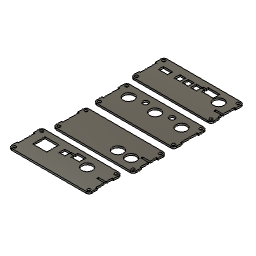
BlinkBoxEndV2v5 (Autodesk Fusion 360 design; units mm, degrees)
Autodesk Fusion 360 part; units mm, degrees
sketch "FrontSketch" plane through (0, 0, 0) normal (0, 1, 0) x (1, 0, 0)
  line L0 (0, 0) -> (92, 0) construction
  line L1 (0, 0) -> (-2.45, 0) construction
  line L2 (94.45, 0) -> (92, 0) construction
  line L3 (-2.45, 8) -> (94.45, 8) construction
  line L4 (94.45, 8) -> (94.45, -31.9) construction
  line L5 (94.45, -31.9) -> (-2.45, -31.9) construction
  line L6 (-2.45, -31.9) -> (-2.45, 8) construction
  line L7 (-2.45, -28.4) -> (1.05, -28.4) construction
  line L8 (1.05, -28.4) -> (1.05, -31.9) construction
  circle A0 centre (1.05, -28.4) radius 1.825
  arc A1 (-2.45, -28.4) -> (1.05, -31.9) centre (1.05, -28.4) ccw
  line L9 (-2.45, -11.95) -> (94.45, -11.95) construction
  line L10 (46, -31.9) -> (46, 8) construction
  arc A2 (90.95, -31.9) -> (94.45, -28.4) centre (90.95, -28.4) ccw
  circle A3 centre (90.95, -28.4) radius 1.825
  circle A4 centre (1.05, 4.5) radius 1.825
  arc A5 (1.05, 8) -> (-2.45, 4.5) centre (1.05, 4.5) ccw
  circle A6 centre (90.95, 4.5) radius 1.825
  arc A7 (94.45, 4.5) -> (90.95, 8) centre (90.95, 4.5) ccw
  line L11 (94.45, 4.5) -> (94.45, -28.4)
  line L12 (90.95, 8) -> (1.05, 8)
  line L13 (-2.45, 4.5) -> (-2.45, -28.4)
  line L14 (1.05, -31.9) -> (90.95, -31.9)
  line L15 (14, 0) -> (14, -6) construction
  circle A8 centre (14, -6) radius 6.5
  line L16 (30, 0) -> (30, -1.5) construction
  circle A9 centre (30, -1.5) radius 3.25
  circle A10 centre (78, -6) radius 6.5
  circle A11 centre (62, -1.5) radius 3.25
  line L17 (46, 0) -> (46, -6) construction
  circle A12 centre (46, -6) radius 6.5
  line L18 (-2.45, -21.8) -> (-0.95, -21.8)
  line L19 (-2.45, -2.1) -> (-0.95, -2.1)
  line L20 (-0.95, -21.8) -> (-0.95, -2.1)
  line L21 (94.45, -21.8) -> (92.95, -21.8)
  line L22 (92.95, -21.8) -> (92.95, -2.1)
  line L23 (94.45, -2.1) -> (92.95, -2.1)
  line L24 (20.5, 8) -> (20.5, -16.9385) construction
  line L25 (26.75, 8) -> (26.75, -12.4751) construction
  dimension "d3" = 92
  dimension "d5" = 39.9
  dimension "d6" = 96.9
  dimension "d7" = 3.5
  dimension "d8" = 3.65
  dimension "d11" = 8
  dimension "d12" = 6
  dimension "d13" = 14
  dimension "d14" = 13
  dimension "d15" = 30
  dimension "d16" = 1.5
  dimension "d17" = 6.5
  dimension "d18" = 6
  dimension "d19" = 13
  dimension "d23" = 1.5
  dimension "d24" = 19.7
  dimension "d25" = 6.25
  constraint coincident L0.start L1.start
  constraint horizontal L0
  constraint parallel L0 L2
  constraint horizontal L3
  constraint vertical L4
  constraint horizontal L5
  constraint vertical L6
  constraint coincident L1.end L6
  constraint coincident L2.start L4
  constraint equal L1 L2
  constraint coincident L6 L7.start
  constraint perpendicular L6 L7
  constraint coincident L5 L8.end
  constraint perpendicular L5 L8
  constraint equal L7 L8
  constraint coincident L7.end L8.start
  constraint midpoint L6 L9.start
  constraint midpoint L4 L9.end
  constraint midpoint L5 L10.start
  constraint midpoint L3 L10.end
  constraint symmetric L7.start L10 A2.end
  constraint symmetric L8.end L10 A2.start
  constraint symmetric A0 L10 A3
  constraint symmetric A1 L10 A2
  constraint symmetric L7.start L9 A5.end
  constraint symmetric L8.end L9 A5.start
  constraint symmetric A0 L9 A4
  constraint symmetric A1 L9 A5
  constraint symmetric L9 A2.end A7.start
  constraint symmetric L9 A2.start A7.end
  constraint symmetric L9 A2 A7
  constraint symmetric L9 A3 A6
  constraint tangent A2 L11
  constraint coincident L0 L15.start
  constraint perpendicular L0 L15
  constraint coincident L15.end A8.centre
  constraint coincident L0 L16.start
  constraint perpendicular L0 L16
  constraint coincident L16.end A9.centre
  constraint symmetric L10 A8 A10
  constraint symmetric L10 A9 A11
  constraint midpoint L0 L17.start
  constraint coincident L10 L17.end
  constraint perpendicular L0 L17
  constraint coincident L17.end A12.centre
  constraint coincident L6 L18.start
  constraint perpendicular L6 L18
  constraint symmetric L9 L18.start L19.start
  constraint symmetric L9 L18.end L19.end
  constraint symmetric L10 L18.start L21.start
  constraint symmetric L10 L18.end L21.end
  constraint symmetric L10 L19.start L23.start
  constraint symmetric L10 L19.end L22.end
  constraint coincident L12 L24.start
  constraint perpendicular L9 L24
  constraint tangent A8 L24
  constraint coincident L12 L25.start
  constraint perpendicular L9 L25
  constraint tangent A9 L25
  measures "d3" distance of L0.start L0.end
  measures "d5" distance of L3.start L5.end
  measures "d6" distance of L4.end L5.end
  measures "d7" distance of L7.end L8.end
  measures "d8" diameter of A0
  measures "d11" distance of L1 L3
  measures "d12" distance of L15.start L15.end
  measures "d13" distance of L0.start L15.start
  measures "d14" diameter of A8
  measures "d15" distance of L0.start L16.start
  measures "d16" distance of L16.start L16.end
  measures "d17" diameter of A9
  measures "d18" distance of L17.start L17.end
  measures "d19" diameter of A12
  measures "d23" distance of L18.start L18.end
  measures "d24" distance of L18.end L19.end
  measures "d25" distance of L24 L25
extrude "Extrude1" add sketch "FrontSketch" against normal blind 2 contours A1 A2 A5 A7 L11 L12 L13 L14 L18 L19 L20 L21 L22 L23 makes body 1
move_body "Move1" bodies 1 to x (1, 0, 0) y (0, 0, -1) z (0, 1, 0) at (0, 6, -10)
extrude "Extrude2" add sketch "FrontSketch" along normal blind 2 separate body contours A1 A2 A5 A7 L11 L12 L13 L14 L18 L19 L20 L21 L22 L23 | A8 | A9 | A11 | A12 makes body 2
move_body "Move2" bodies 2 to x (1, 0, 0) y (0, 0, -1) z (0, 1, 0) at (0, 8, -8)
move_body "Move3" bodies 2 to x (1, 0, 0) y (0, 1, 0) z (0, 0, 1) at (0, 41, 0)
sketch "BackSketch" plane through (0, 0, 0) normal (0, 1, 0) x (1, 0, 0)
  circle A0 centre (-2.9196, -31.4778) radius 1.825
  line L0 (16.5304, 4.9222) -> (16.5304, -16.9386) construction
  line L1 (90.4804, -5.1778) -> (88.9804, -5.1778)
  line L2 (42.0304, -34.9778) -> (42.0304, 4.9222) construction
  circle A1 centre (74.0304, -9.0778) radius 6.5
  line L3 (-3.9696, -3.0778) -> (-6.4196, -3.0778) construction
  line L4 (88.9804, -24.8778) -> (88.9804, -5.1778)
  line L5 (-4.9196, -24.8778) -> (-4.9196, -5.1778)
  line L6 (-3.9696, -3.0778) -> (88.0304, -3.0778) construction
  line L7 (-6.4196, -24.8778) -> (-4.9196, -24.8778)
  line L8 (-6.4196, -5.1778) -> (-4.9196, -5.1778)
  circle A2 centre (86.9804, -31.4778) radius 1.825
  arc A3 (90.4804, 1.4222) -> (86.9804, 4.9222) centre (86.9804, 1.4222) ccw
  line L9 (86.9804, 4.9222) -> (-2.9196, 4.9222)
  line L10 (90.4804, -24.8778) -> (88.9804, -24.8778)
  line L11 (90.4804, 4.9222) -> (90.4804, -34.9778) construction
  arc A4 (86.9804, -34.9778) -> (90.4804, -31.4778) centre (86.9804, -31.4778) ccw
  circle A5 centre (10.0304, -9.0778) radius 6.5 construction
  line L12 (90.4804, 1.4222) -> (90.4804, -31.4778)
  arc A6 (-2.9196, 4.9222) -> (-6.4196, 1.4222) centre (-2.9196, 1.4222) ccw
  line L13 (-6.4196, -34.9778) -> (-6.4196, 4.9222) construction
  circle A7 centre (-2.9196, 1.4222) radius 1.825
  line L14 (-6.4196, -15.0278) -> (90.4804, -15.0278) construction
  line L15 (-2.9196, -34.9778) -> (86.9804, -34.9778)
  line L16 (10.0304, -3.0778) -> (10.0304, -9.0778) construction
  circle A8 centre (86.9804, 1.4222) radius 1.825
  line L17 (-2.9196, -31.4778) -> (-2.9196, -34.9778) construction
  line L18 (-6.4196, 1.4222) -> (-6.4196, -31.4778)
  line L19 (-6.4196, 4.9222) -> (90.4804, 4.9222) construction
  arc A9 (-6.4196, -31.4778) -> (-2.9196, -34.9778) centre (-2.9196, -31.4778) ccw
  line L20 (-6.4196, -31.4778) -> (-2.9196, -31.4778) construction
  line L21 (90.4804, -34.9778) -> (-6.4196, -34.9778) construction
  line L22 (90.4804, -3.0778) -> (88.0304, -3.0778) construction
  line L23 (59.4804, -3.0778) -> (59.4804, -4.0778) construction
  line L24 (66.4804, -0.0778) -> (52.4804, -0.0778)
  line L25 (52.4804, -0.0778) -> (52.4804, -8.0778)
  line L26 (52.4804, -8.0778) -> (66.4804, -8.0778)
  line L27 (66.4804, -8.0778) -> (66.4804, -0.0778)
  line L28 (66.4804, -0.0778) -> (52.4804, -8.0778) construction
  line L29 (52.4804, -0.0778) -> (66.4804, -8.0778) construction
  line L30 (45.0304, -3.0778) -> (45.0304, -7.0778) construction
  line L31 (48.5304, -3.5778) -> (41.5304, -3.5778)
  line L32 (41.5304, -3.5778) -> (41.5304, -10.5778)
  line L33 (41.5304, -10.5778) -> (48.5304, -10.5778)
  line L34 (48.5304, -10.5778) -> (48.5304, -3.5778)
  line L35 (48.5304, -3.5778) -> (41.5304, -10.5778) construction
  line L36 (41.5304, -3.5778) -> (48.5304, -10.5778) construction
  line L37 (45.0304, -7.0778) -> (35.0304, -7.0778) construction
  line L38 (35.0304, -7.0778) -> (25.0304, -7.0778) construction
  line L39 (38.5304, -3.5778) -> (31.5304, -3.5778)
  line L40 (31.5304, -3.5778) -> (31.5304, -10.5778)
  line L41 (31.5304, -10.5778) -> (38.5304, -10.5778)
  line L42 (38.5304, -10.5778) -> (38.5304, -3.5778)
  line L43 (38.5304, -3.5778) -> (31.5304, -10.5778) construction
  line L44 (31.5304, -3.5778) -> (38.5304, -10.5778) construction
  line L45 (28.5304, -3.5778) -> (21.5304, -3.5778)
  line L46 (21.5304, -3.5778) -> (21.5304, -10.5778)
  line L47 (21.5304, -10.5778) -> (28.5304, -10.5778)
  line L48 (28.5304, -10.5778) -> (28.5304, -3.5778)
  line L49 (28.5304, -3.5778) -> (21.5304, -10.5778) construction
  line L50 (21.5304, -3.5778) -> (28.5304, -10.5778) construction
  line L51 (10.0304, -3.0778) -> (-3.9696, -3.0778) construction
  line L52 (8.5304, -3.0778) -> (8.5304, -8.0778) construction
  line L53 (8.5304, -3.0778) -> (-3.9696, -3.0778)
  line L54 (14.0304, -5.0778) -> (3.0304, -5.0778)
  line L55 (3.0304, -5.0778) -> (3.0304, -11.0778)
  line L56 (3.0304, -11.0778) -> (14.0304, -11.0778)
  line L57 (14.0304, -11.0778) -> (14.0304, -5.0778)
  line L58 (14.0304, -5.0778) -> (3.0304, -11.0778) construction
  line L59 (3.0304, -5.0778) -> (14.0304, -11.0778) construction
  line L60 (88.9804, -20.8488) -> (79.9804, -20.8488)
  line L61 (79.9804, -20.8488) -> (79.9804, -18.8488)
  line L62 (79.9804, -18.8488) -> (88.9804, -18.8488)
  line L63 (88.9804, -18.8488) -> (88.9804, -20.8488)
  line L64 (49.5904, -20.979) -> (74.5904, -20.979)
  line L65 (49.5904, -20.979) -> (62.0904, -13.0411)
  line L66 (62.0904, -13.0411) -> (74.5904, -20.979)
  line L67 (48.5304, -4.4715) -> (52.4804, -4.4715)
  line L68 (52.4804, -4.4715) -> (52.4804, -2.4715)
  line L69 (52.4804, -2.4715) -> (48.5304, -2.4715)
  line L70 (48.5304, -2.4715) -> (48.5304, -4.4715)
  point P0 (-3.9696, -3.0778)
  point P1 (59.4804, -4.0778)
  point P2 (45.0304, -7.0778)
  point P3 (35.0304, -7.0778)
  point P4 (25.0304, -7.0778)
  point P5 (8.5304, -8.0778)
  point P6 (60.5604, -18.5803)
  dimension "d32" = 92
  dimension "d33" = 39.9
  dimension "d34" = 96.9
  dimension "d35" = 3.5
  dimension "d36" = 3.65
  dimension "d37" = 8
  dimension "d38" = 6
  dimension "d40" = 13
  dimension "d46" = 1.5
  dimension "d47" = 19.7
  dimension "d49" = 8
  dimension "d50" = 14
  dimension "d51" = 1
  dimension "d52" = 24
  dimension "d53" = 3
  dimension "d54" = 4
  dimension "d55" = 7
  dimension "d56" = 7
  dimension "d57" = 10
  dimension "d58" = 10
  dimension "d59" = 7
  dimension "d60" = 7
  dimension "d61" = 7
  dimension "d62" = 7
  dimension "d78" = 14
  dimension "d79" = 12.5
  dimension "d80" = 5
  dimension "d81" = 6
  dimension "d82" = 11
  dimension "d83" = 9
  dimension "d84" = 2
  dimension "d88" = 25
  dimension "d92" = 2
  constraint coincident P0 L3.start
  constraint horizontal L6
  constraint parallel L6 L22
  constraint horizontal L19
  constraint vertical L11
  constraint horizontal L21
  constraint vertical L13
  constraint coincident L3.end L13
  constraint coincident L22.start L11
  constraint equal L3 L22
  constraint coincident L18.end L13
  constraint perpendicular L13 L20
  constraint coincident L15.start L21
  constraint perpendicular L17 L21
  constraint equal L17 L20
  constraint coincident A0.centre L17.start
  constraint midpoint L14.start L13
  constraint midpoint L14.end L11
  constraint midpoint L2.start L21
  constraint midpoint L2.end L19
  constraint symmetric A4.end L18.end L2
  constraint symmetric A4.start L15.start L2
  constraint symmetric A0 L2 A2
  constraint symmetric L2 A4 A9
  constraint symmetric L18.end A6.end L14
  constraint symmetric L15.start L9.end L14
  constraint symmetric A0 A7 L14
  constraint symmetric A6 L14 A9
  constraint symmetric A4.end A3.start L14
  constraint symmetric A4.start A3.end L14
  constraint symmetric A3 A4 L14
  constraint symmetric A2 L14 A8
  constraint tangent A4 L12
  constraint coincident L16.start L6
  constraint perpendicular L6 L16
  constraint coincident A5.centre L16.end
  constraint symmetric L2 A1 A5
  constraint coincident L7.start L13
  constraint perpendicular L7 L13
  constraint symmetric L8.start L7.start L14
  constraint symmetric L5.end L5.start L14
  constraint symmetric L10.start L7.start L2
  constraint symmetric L4.start L5.start L2
  constraint symmetric L1.start L8.start L2
  constraint symmetric L5.end L1.end L2
  constraint coincident L0.start L9
  constraint perpendicular L0 L14
  constraint tangent L0 A5
  constraint coincident L6 L23.start
  constraint perpendicular L6 L23
  constraint horizontal L24
  constraint perpendicular L24 L25
  constraint parallel L24 L26
  constraint parallel L25 L27
  constraint coincident L28 P1
  constraint coincident L29 P1
  constraint coincident P1 L23.end
  constraint coincident L6 L30.start
  constraint perpendicular L6 L30
  constraint horizontal L31
  constraint perpendicular L31 L32
  constraint parallel L31 L33
  constraint parallel L32 L34
  constraint coincident L35 P2
  constraint coincident L36 P2
  constraint coincident P2 L30.end
  constraint perpendicular L30 L37
  constraint parallel L37 L38
  constraint horizontal L39
  constraint perpendicular L39 L40
  constraint parallel L39 L41
  constraint parallel L40 L42
  constraint coincident L43 P3
  constraint coincident L44 P3
  constraint coincident P3 L37.end
  constraint horizontal L45
  constraint perpendicular L45 L46
  constraint parallel L45 L47
  constraint parallel L46 L48
  constraint coincident L49 P4
  constraint coincident L50 P4
  constraint coincident P4 L38.end
  constraint coincident L51 L52.start
  constraint perpendicular L51 L52
  constraint horizontal L54
  constraint perpendicular L54 L55
  constraint parallel L54 L56
  constraint parallel L55 L57
  constraint coincident L58 P5
  constraint coincident L59 P5
  constraint coincident P5 L52.end
  constraint horizontal L60
  constraint vertical L61
  constraint horizontal L62
  constraint vertical L63
  constraint coincident L4 L60.start
  constraint horizontal L64
  constraint equal L65 L66
  constraint horizontal L67
  constraint vertical L68
  constraint horizontal L69
  constraint vertical L70
  constraint coincident L25 L68.end
  constraint coincident L34 L67.start
  measures "d32" distance of L6.end P0
  measures "d33" distance of L13.end L13.start
  measures "d34" distance of L13.start L11.end
  measures "d35" distance of L15.start A0.centre
  measures "d36" diameter of A0
  measures "d37" distance of L3 L19
  measures "d38" distance of L16.start A5.centre
  measures "d40" diameter of A5
  measures "d46" distance of L5.start L7.start
  measures "d47" distance of L5.end L5.start
  measures "d49" distance of L24.start L26.end
  measures "d50" distance of L24.start L24.end
  measures "d51" distance of L23.start P1
  measures "d52" distance of L11 L27
  measures "d53" distance of L2 L30
  measures "d54" distance of L30.start P2
  measures "d55" distance of L32.end L33.end
  measures "d56" distance of L31.start L33.end
  measures "d57" distance of P2 P3
  measures "d58" distance of P3 P4
  measures "d59" distance of L39.start L41.end
  measures "d60" distance of L40.end L41.end
  measures "d61" distance of L45.start L47.end
  measures "d62" distance of L46.end L47.end
  measures "d78" distance of L16.start P0
  measures "d79" distance of L52.start P0
  measures "d80" distance of L52.start P5
  measures "d81" distance of L54.end L55.end
  measures "d82" distance of L55.end L56.end
  measures "d83" distance of L60.start L60.end
  measures "d84" distance of L60.end L61.end
  measures "d88" distance of L64.start L64.end
  measures "d92" distance of L67 L69
extrude "Extrude3" add sketch "BackSketch" along normal blind 2 separate body contours L1 L4 L5 L7 L8 A3 L9 L10 A4 L12 A6 L15 L18 A9 L60 L61 L62 | L64 L65 L66 makes body 3
extrude "Extrude4" add sketch "BackSketch" along normal blind 2 separate body contours L64 L65 L66 makes body 4
combine "Combine1" operation add target body 3 tool bodies 4
move_body "Move4" bodies 3 to x (1, 0, 0) y (0, 0, -1) z (0, 1, 0) at (0, 6.9222, -2.9222)
move_face "MoveFace1" by (0, 37, 0) 1 faces at (41.8637, 33.7667, -2.9222) on bodies 3
move_body "Move5" bodies 3 to x (1, 0, 0) y (0, 1, 0) z (0, 0, 1) at (0, 45, 0)
delete_body "RemoveBody1" bodies 2
move_body "Move6" bodies 1 to x (1, 0, 0) y (0, -1, 0) z (0, 0, -1) at (0, 75.8, -16)
move_body "Move7" bodies 3 to x (1, 0, 0) y (0, -1, 0) z (0, 0, -1) at (0, 173.8, -5.8444)
sketch "ClockFrontSketc" plane through (0, 0, 0) normal (0, 1, 0) x (1, 0, 0)
  line L0 (-3.191, -12.6593) -> (93.709, -12.6593) construction
  line L1 (0.309, -32.6093) -> (90.209, -32.6093)
  circle A0 centre (45.259, -6.7093) radius 6.5
  line L2 (45.259, -32.6093) -> (45.259, 7.2907) construction
  line L3 (90.209, 7.2907) -> (0.309, 7.2907)
  line L4 (45.259, -0.7093) -> (45.259, -6.7093) construction
  line L5 (93.709, -32.6093) -> (-3.191, -32.6093) construction
  line L6 (-0.741, -0.7093) -> (91.259, -0.7093) construction
  line L7 (-3.191, 7.2907) -> (93.709, 7.2907) construction
  line L8 (93.709, -22.5093) -> (92.209, -22.5093)
  circle A1 centre (90.209, -29.1093) radius 1.825
  line L9 (13.259, -0.7093) -> (13.259, -6.7093) construction
  arc A2 (90.209, -32.6093) -> (93.709, -29.1093) centre (90.209, -29.1093) ccw
  circle A3 centre (0.309, -29.1093) radius 1.825
  line L10 (93.709, -0.7093) -> (91.259, -0.7093) construction
  circle A4 centre (77.259, -6.7093) radius 6.5
  line L11 (-3.191, -29.1093) -> (0.309, -29.1093) construction
  line L12 (-3.191, 3.7907) -> (-3.191, -29.1093)
  line L13 (92.209, -22.5093) -> (92.209, -2.8093)
  line L14 (-1.691, -22.5093) -> (-1.691, -2.8093)
  arc A5 (93.709, 3.7907) -> (90.209, 7.2907) centre (90.209, 3.7907) ccw
  circle A6 centre (13.259, -6.7093) radius 6.5
  line L15 (-3.191, -2.8093) -> (-1.691, -2.8093)
  line L16 (93.709, 7.2907) -> (93.709, -32.6093) construction
  line L17 (0.309, -29.1093) -> (0.309, -32.6093) construction
  circle A7 centre (0.309, 3.7907) radius 1.825
  arc A8 (0.309, 7.2907) -> (-3.191, 3.7907) centre (0.309, 3.7907) ccw
  line L18 (93.709, -2.8093) -> (92.209, -2.8093)
  line L19 (-3.191, -22.5093) -> (-1.691, -22.5093)
  arc A9 (-3.191, -29.1093) -> (0.309, -32.6093) centre (0.309, -29.1093) ccw
  line L20 (-3.191, -32.6093) -> (-3.191, 7.2907) construction
  line L21 (-0.741, -0.7093) -> (-3.191, -0.7093) construction
  circle A10 centre (90.209, 3.7907) radius 1.825
  line L22 (93.709, 3.7907) -> (93.709, -29.1093)
  line L23 (13.259, -6.7093) -> (45.259, -6.7093) construction
  circle A11 centre (29.259, -6.7093) radius 6.5
  line L24 (93.709, -12.6593) -> (-3.191, -12.6593) construction
  circle A12 centre (61.259, -6.7093) radius 6.5
  line L25 (83.209, -14.6593) -> (92.209, -14.6593)
  line L26 (92.209, -14.6593) -> (92.209, -12.6593)
  line L27 (92.209, -12.6593) -> (83.209, -12.6593)
  line L28 (83.209, -12.6593) -> (83.209, -14.6593)
  point P0 (-0.741, -0.7093)
  dimension "d93" = 92
  dimension "d94" = 39.9
  dimension "d95" = 96.9
  dimension "d96" = 3.5
  dimension "d97" = 3.65
  dimension "d98" = 8
  dimension "d99" = 6
  dimension "d100" = 14
  dimension "d101" = 13
  dimension "d105" = 6
  dimension "d106" = 13
  dimension "d107" = 1.5
  dimension "d108" = 19.7
  dimension "d110" = 13
  dimension "d155" = 9
  dimension "d156" = 2
  constraint coincident P0 L6.start
  constraint horizontal L6
  constraint parallel L6 L10
  constraint horizontal L7
  constraint vertical L16
  constraint horizontal L5
  constraint vertical L20
  constraint coincident L21.end L20
  constraint coincident L10.start L16
  constraint equal L10 L21
  constraint coincident L11.start L20
  constraint perpendicular L11 L20
  constraint coincident L1.start L5
  constraint perpendicular L5 L17
  constraint equal L11 L17
  constraint coincident A3.centre L11.end
  constraint midpoint L0.start L20
  constraint midpoint L0.end L16
  constraint midpoint L2.start L5
  constraint midpoint L2.end L7
  constraint symmetric A2.end L11.start L2
  constraint symmetric L1.start L1.end L2
  constraint symmetric L2 A1 A3
  constraint symmetric L2 A2 A9
  constraint symmetric L11.start L12.start L0
  constraint symmetric L1.start L3.end L0
  constraint symmetric L0 A3 A7
  constraint symmetric L0 A8 A9
  constraint symmetric A2.end A5.start L0
  constraint symmetric L3.start L1.end L0
  constraint symmetric L0 A2 A5
  constraint symmetric L0 A1 A10
  constraint tangent A2 L22
  constraint coincident L9.start L6
  constraint perpendicular L6 L9
  constraint coincident L9.end A6.centre
  constraint symmetric L2 A4 A6
  constraint midpoint L4.start L6
  constraint coincident A0.centre L2
  constraint perpendicular L4 L6
  constraint coincident A0.centre L4.end
  constraint coincident L19.start L20
  constraint perpendicular L19 L20
  constraint symmetric L19.start L15.start L0
  constraint symmetric L14.start L14.end L0
  constraint symmetric L8.start L19.start L2
  constraint symmetric L14.start L8.end L2
  constraint symmetric L15.start L18.start L2
  constraint symmetric L13.end L14.end L2
  constraint midpoint L23 A11.centre
  constraint symmetric L0.start L2 L0.end
  constraint symmetric L0.end L2 L0.start
  constraint symmetric L2 A11 A12
  constraint horizontal L25
  constraint vertical L26
  constraint horizontal L27
  constraint vertical L28
  constraint midpoint L13 L26.end
  measures "d93" distance of P0 L6.end
  measures "d94" distance of L5.end L7.start
  measures "d95" distance of L5.end L5.start
  measures "d96" distance of A3.centre L1.start
  measures "d97" diameter of A3
  measures "d98" distance of L7 L21
  measures "d99" distance of L9.start L9.end
  measures "d100" distance of L9.start P0
  measures "d101" diameter of A6
  measures "d105" distance of L4.start A0.centre
  measures "d106" diameter of A0
  measures "d107" distance of L14.start L19.start
  measures "d108" distance of L14.start L14.end
  measures "d110" diameter of A11
  measures "d155" distance of L25.start L25.end
  measures "d156" distance of L25.start L27.end
extrude "Extrude5" add sketch "ClockFrontSketc" along normal blind 2 separate body contours L1 L3 L8 A2 L12 L13 L14 A5 L15 A8 L18 L19 A9 L22 L25 L27 L28 | A0 | A6 | A11 makes body 5
move_body "Move8" bodies 5 to x (1, 0, 0) y (0, 0, 1) z (0, -1, 0) at (0, 22, -8)
sketch "ClockBackSketch" plane through (0, 0, 0) normal (0, 1, 0) x (1, 0, 0)
  line L0 (52.0304, -14.044) -> (52.0304, -6.044)
  line L1 (-3.9696, -9.044) -> (88.0304, -9.044) construction
  line L2 (37.0304, -9.544) -> (30.0304, -16.544) construction
  line L3 (86.9804, -1.044) -> (-2.9196, -1.044)
  line L4 (30.0304, -9.544) -> (30.0304, -16.544)
  line L5 (42.0304, -6.044) -> (42.0304, -14.044)
  line L6 (42.0304, -40.944) -> (42.0304, -1.044) construction
  line L7 (42.0304, -6.044) -> (52.0304, -14.044) construction
  line L8 (30.0304, -9.544) -> (37.0304, -16.544) construction
  line L9 (30.0304, -16.544) -> (37.0304, -16.544)
  line L10 (33.5304, -9.044) -> (33.5304, -13.044) construction
  line L11 (52.0304, -6.044) -> (42.0304, -14.044) construction
  line L12 (52.0304, -6.044) -> (42.0304, -6.044)
  line L13 (-2.9196, -40.944) -> (86.9804, -40.944)
  line L14 (-6.4196, -1.044) -> (90.4804, -1.044) construction
  line L15 (90.4804, -40.944) -> (-6.4196, -40.944) construction
  line L16 (47.0304, -9.044) -> (47.0304, -10.044) construction
  line L17 (42.0304, -4.4715) -> (42.0304, -2.4715)
  line L18 (37.0304, -9.544) -> (30.0304, -9.544)
  line L19 (5.0304, -8.544) -> (22.0304, -23.544) construction
  line L20 (22.0304, -8.544) -> (5.0304, -23.544) construction
  line L21 (13.5304, -9.044) -> (-3.9696, -9.044)
  line L22 (5.0304, -23.544) -> (22.0304, -23.544)
  circle A0 centre (86.9804, -4.544) radius 1.825
  line L23 (88.9804, -20.8488) -> (79.9804, -20.8488)
  line L24 (7.3292, -9.044) -> (-3.9696, -9.044) construction
  line L25 (42.0304, -14.044) -> (52.0304, -14.044)
  line L26 (22.0304, -8.544) -> (5.0304, -8.544)
  line L27 (90.4804, -30.844) -> (88.9804, -30.844)
  line L28 (-6.4196, -4.544) -> (-6.4196, -37.444)
  line L29 (37.0304, -16.544) -> (37.0304, -9.544)
  line L30 (90.4804, -1.044) -> (90.4804, -40.944) construction
  line L31 (88.9804, -18.8488) -> (88.9804, -20.8488)
  arc A1 (-6.4196, -37.444) -> (-2.9196, -40.944) centre (-2.9196, -37.444) ccw
  circle A2 centre (86.9804, -37.444) radius 1.825
  arc A3 (90.4804, -4.544) -> (86.9804, -1.044) centre (86.9804, -4.544) ccw
  line L32 (5.0304, -8.544) -> (5.0304, -23.544)
  line L33 (90.4804, -4.544) -> (90.4804, -37.444)
  line L34 (90.4804, -11.144) -> (88.9804, -11.144)
  line L35 (90.4804, -9.044) -> (88.0304, -9.044) construction
  line L36 (22.0304, -23.544) -> (22.0304, -8.544)
  line L37 (88.9804, -30.844) -> (88.9804, -11.144)
  line L38 (13.5304, -9.044) -> (13.5304, -16.044) construction
  line L39 (-6.4196, -37.444) -> (-2.9196, -37.444) construction
  line L40 (79.9804, -20.8488) -> (79.9804, -18.8488)
  line L41 (79.9804, -18.8488) -> (88.9804, -18.8488)
  arc A4 (86.9804, -40.944) -> (90.4804, -37.444) centre (86.9804, -37.444) ccw
  arc A5 (-2.9196, -1.044) -> (-6.4196, -4.544) centre (-2.9196, -4.544) ccw
  line L42 (16.5304, -1.044) -> (16.5304, -16.9386) construction
  line L43 (-6.4196, -30.844) -> (-4.9196, -30.844)
  line L44 (-2.9196, -37.444) -> (-2.9196, -40.944) construction
  circle A6 centre (-2.9196, -4.544) radius 1.825
  line L45 (-6.4196, -11.144) -> (-4.9196, -11.144)
  line L46 (-3.9696, -9.044) -> (-6.4196, -9.044) construction
  circle A7 centre (-2.9196, -37.444) radius 1.825
  line L47 (-6.4196, -40.944) -> (-6.4196, -1.044) construction
  line L48 (-4.9196, -30.844) -> (-4.9196, -11.144)
  line L49 (-6.4196, -20.994) -> (90.4804, -20.994) construction
  circle A8 centre (62.4804, -15.044) radius 6.5
  line L50 (62.4804, -15.044) -> (62.4804, -9.044) construction
  line L51 (62.4804, -15.044) -> (90.4804, -15.044) construction
  line L52 (37.0304, -11.044) -> (42.0304, -11.044)
  line L53 (42.0304, -11.044) -> (42.0304, -9.044)
  line L54 (42.0304, -9.044) -> (37.0304, -9.044)
  line L55 (37.0304, -9.044) -> (37.0304, -11.044)
  point P0 (47.0304, -10.044)
  point P1 (33.5304, -13.044)
  point P2 (-3.9696, -9.044)
  point P3 (60.5604, -18.5803)
  point P4 (13.5304, -16.044)
  dimension "d113" = 92
  dimension "d114" = 39.9
  dimension "d115" = 96.9
  dimension "d116" = 3.5
  dimension "d117" = 3.65
  dimension "d118" = 8
  dimension "d121" = 1.5
  dimension "d122" = 19.7
  dimension "d123" = 8
  dimension "d125" = 1
  dimension "d128" = 4
  dimension "d129" = 7
  dimension "d130" = 7
  dimension "d138" = 17.5
  dimension "d139" = 7
  dimension "d140" = 15
  dimension "d141" = 17
  dimension "d142" = 9
  dimension "d143" = 2
  dimension "d146" = 6
  dimension "d147" = 28
  dimension "d148" = 13
  dimension "d149" = 8
  dimension "d150" = 5
  dimension "d151" = 10
  dimension "d152" = 2
  constraint coincident P2 L1.start
  constraint horizontal L1
  constraint parallel L1 L35
  constraint horizontal L14
  constraint vertical L30
  constraint horizontal L15
  constraint vertical L47
  constraint coincident L46.end L47
  constraint coincident L35.start L30
  constraint equal L35 L46
  constraint coincident L28.end L47
  constraint perpendicular L39 L47
  constraint coincident L13.start L15
  constraint perpendicular L15 L44
  constraint equal L39 L44
  constraint coincident A1.centre L39.end
  constraint midpoint L49.start L47
  constraint midpoint L49.end L30
  constraint midpoint L6.start L15
  constraint midpoint L6.end L14
  constraint symmetric L28.end L33.end L6
  constraint symmetric L13.end L13.start L6
  constraint symmetric L6 A2 A7
  constraint symmetric L6 A1 A4
  constraint symmetric L28.end L28.start L49
  constraint symmetric L3.end L13.start L49
  constraint symmetric A6 A7 L49
  constraint symmetric A1 A5 L49
  constraint symmetric L33.end A3.start L49
  constraint symmetric L3.start L13.end L49
  constraint symmetric A3 A4 L49
  constraint symmetric A0 A2 L49
  constraint tangent L33 A4
  constraint coincident L24.start L1
  constraint coincident L43.start L47
  constraint perpendicular L43 L47
  constraint symmetric L43.start L45.start L49
  constraint symmetric L43.end L45.end L49
  constraint symmetric L27.start L43.start L6
  constraint symmetric L27.end L43.end L6
  constraint symmetric L34.start L45.start L6
  constraint symmetric L34.end L45.end L6
  constraint coincident L42.start L3
  constraint perpendicular L42 L49
  constraint coincident L16.start L1
  constraint perpendicular L1 L16
  constraint horizontal L12
  constraint perpendicular L5 L12
  constraint parallel L12 L25
  constraint parallel L0 L5
  constraint coincident P0 L11
  constraint coincident P0 L7
  constraint coincident P0 L16.end
  constraint coincident L10.start L1
  constraint perpendicular L1 L10
  constraint horizontal L18
  constraint perpendicular L4 L18
  constraint parallel L9 L18
  constraint parallel L4 L29
  constraint coincident P1 L2
  constraint coincident P1 L8
  constraint coincident P1 L10.end
  constraint coincident L21.start L24
  constraint perpendicular L24 L38
  constraint horizontal L26
  constraint perpendicular L26 L32
  constraint parallel L22 L26
  constraint parallel L32 L36
  constraint coincident P4 L20
  constraint coincident P4 L19
  constraint coincident P4 L38.end
  constraint horizontal L23
  constraint vertical L40
  constraint horizontal L41
  constraint vertical L31
  constraint coincident L23.start L37
  constraint vertical L17
  constraint coincident L17.end L5
  constraint coincident A8.centre L50.start
  constraint coincident L1 L50.end
  constraint perpendicular L1 L50
  constraint coincident L30 L51.end
  constraint perpendicular L30 L51
  constraint horizontal L52
  constraint vertical L53
  constraint horizontal L54
  constraint vertical L55
  constraint midpoint L1 L53.end
  constraint coincident L29 L52.start
  measures "d113" distance of P2 L1.end
  measures "d114" distance of L15.end L14.start
  measures "d115" distance of L15.end L15.start
  measures "d116" distance of A1.centre L13.start
  measures "d117" diameter of A7
  measures "d118" distance of L14 L46
  measures "d121" distance of L43.end L43.start
  measures "d122" distance of L43.end L45.end
  measures "d123" distance of L0.start L0.end
  measures "d125" distance of P0 L16.start
  measures "d128" distance of P1 L10.start
  measures "d129" distance of L8.end L2.end
  measures "d130" distance of L8.end L2.start
  measures "d138" distance of P2 L21.start
  measures "d139" distance of L21.start P4
  measures "d140" distance of L19.start L20.end
  measures "d141" distance of L19.end L20.end
  measures "d142" distance of L23.start L23.end
  measures "d143" distance of L40.end L23.end
  measures "d146" distance of A8.centre L50.end
  measures "d147" distance of A8.centre L51.end
  measures "d148" diameter of A8
  measures "d149" distance of L4 L36
  measures "d150" distance of L5 L29
  measures "d151" distance of L5.start L0.end
  measures "d152" distance of L1 L52
extrude "Extrude6" add sketch "ClockBackSketch" along normal blind 2 separate body contours L3 L13 L23 L27 L28 A1 A3 L33 L34 L37 L40 L41 A4 A5 L43 L45 L48 makes body 6
move_body "Move9" bodies 6 to x (1, 0, 0) y (0, 0, 1) z (0, -1, 0) at (0, -19.956, -7.956)
move_body "Move10" bodies 3 to x (1, 0, 0) y (0, 1, 0) z (0, 0, 1) at (0, 0, -5)
move_body "Move11" bodies 5 to x (1, 0, 0) y (0, -1, 0) z (0, 0, -1) at (0, 18.7814, -16)
named bodies: "FrontPlate", "BackPlate", "BackPlate2", "ClockFrontPlate", "ClockBackPlate"
